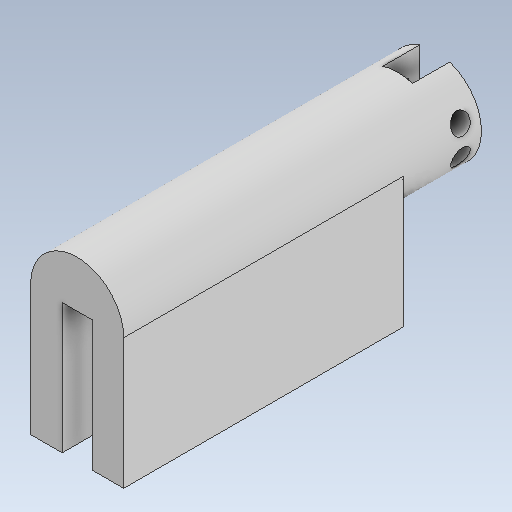
# Autodesk Inventor part: Fahnenhalter
Saved by Autodesk Inventor 2020.3 (Build 243373010, 373A)
## iProperties
Created: 2020-10-20
Part Number: Fahnenhalter
Material: Generisch
Document SubType Name: Modeling
Designer: Stefan
Density: 1 g/cm^3
Appearance: Vorgabe
Author: Stefan
Autodesk Inventor part; units mm, degrees
ref_plane "YZ Plane" through (0, 0, 0) normal (1, 0, 0) x (0, 1, 0)
ref_plane "XZ Plane" through (0, 0, 0) normal (0, 1, 0) x (-1, 0, 0)
ref_plane "XY Plane" through (0, 0, 0) normal (0, 0, 1) x (1, 0, 0)
sketch "Skizze1" plane through (0, 0, 0) normal (0, 0, 1) x (1, 0, 0)
  circle A0 centre (0, 0) radius 12.5
  dimension "d0" = 25
  constraints: 1 centre point, 1 coincident
  measures "d0" diameter of A0
extrude "Extrusion1" add sketch "Skizze1" along normal blind 86
sketch "Skizze3" plane through (0, 0, 86) normal (0, 0, 1) x (1, 0, 0)
  circle A0 centre (0, 0) radius 12.5 projected
  line L0 (-12.5, 0) -> (12.5, 0)
  line L1 (12.5, 0) -> (12.5, -35)
  line L2 (12.5, -35) -> (-12.5, -35)
  line L3 (-12.5, -35) -> (-12.5, 0)
  dimension "d4" = 35
  constraints: 8 end point, 2 parallel, 1 horizontal, 1 perpendicular, 2 other
  measures "d4" distance of L0.end L1.end
extrude "Extrusion2" add sketch "Skizze3" against normal blind 75 contours L1 L2 L3 A0
sketch "Skizze4" plane through (0, 0, 86) normal (0, 0, 1) x (1, 0, 0)
  line L0 (-4, -35.0592) -> (4, -35.0592)
  line L1 (4, -35.0592) -> (4, -0.0592)
  line L2 (4, -0.0592) -> (-4, -0.0592)
  line L3 (-4, -0.0592) -> (-4, -35.0592)
  line L4 (-12.5, 0) -> (-12.5, -35) projected
  line L5 (12.5, -35) -> (12.5, 0) projected
  point P0 (0, 0)
  dimension "d7" = 8
  dimension "d8" = 35
  dimension "d9" = 8.5
  dimension "d10" = 8.5
  constraints: 8 end point, 2 parallel, 1 horizontal, 1 perpendicular
  measures "d7" distance of L2.end L1.end
  measures "d8" distance of L1.end L0.end
  measures "d9" distance between parallel lines of L4 L3
  measures "d10" distance between parallel lines of L5 L1
extrude "Extrusion3" cut sketch "Skizze4" against normal up to surface (75 mm away)
sketch "Skizze5" plane through (0, 0, 0) normal (0, 0, -1) x (-1, 0, 0)
  line L0 (-4, 11.8427) -> (4, 11.8427)
  line L1 (4, 11.8427) -> (4, -11.8427)
  line L2 (4, -11.8427) -> (-4, -11.8427)
  line L3 (-4, -11.8427) -> (-4, 11.8427)
  circle A0 centre (0, 0) radius 12.5
  dimension "d13" = 8
  dimension "d14" = 4
  dimension "d16" = 25
  constraints: 8 end point, 2 parallel, 1 centre point, 1 coincident, 1 horizontal, 1 perpendicular
  measures "d13" distance of L0.start L0.end
  measures "d14" distance from line of point (0, 0) L3
  measures "d16" diameter of A0
extrude "Extrusion4" add sketch "Skizze5" along normal blind 10 contours L3 A0 | A0 L1
sketch "Skizze6" plane through (4, -11.8427, 0) normal (-1, 0, 0) x (0, 0, 1)
  circle A0 centre (-5, 8) radius 2.525
  line L0 (-10, 23.6854) -> (-10, 0) projected
  circle A1 centre (-5, 15.6854) radius 2.525
  line L1 (0, 23.6854) -> (-10, 23.6854) projected
  line L2 (0, 0) -> (-10, 0) projected
  point P0 (0, 11.8427)
  dimension "d19" = 5.05
  dimension "d20" = 5
  dimension "d21" = 5.05
  dimension "d22" = 0
  dimension "d23" = 8
  dimension "d24" = 8
  dimension "d25" = 7.6854
  constraints: 2 centre point
  measures "d19" diameter of A0
  measures "d20" distance from line of A0.centre L0
  measures "d21" diameter of A1
  measures "d22" horizontal distance of A0.centre A1.centre
  measures "d23" distance from line of L1 A1.centre
  measures "d24" distance from line of L2 A0.centre
  measures "d25" distance of A0.centre A1.centre
extrude "Extrusion5" cut sketch "Skizze6" along normal mid plane 500
